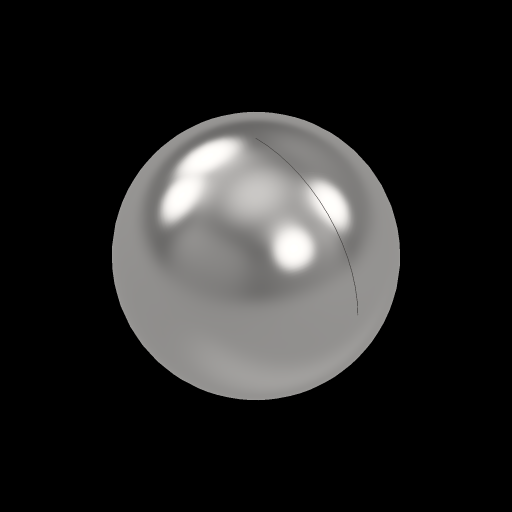
# Autodesk Inventor part: Ball
Saved by Autodesk Inventor 2024 (Build 280153000, 153)
## iProperties
Created: 2023-11-09
Part Number: Ball
Material: Steel, Alloy
Document SubType Name: Modeling
Designer: Admin
Density: 7.73 g/cm^3
Appearance: Semi-Polished
Author: Admin
Autodesk Inventor part; units mm, degrees
ref_plane "YZ Plane" through (0, 0, 0) normal (1, 0, 0) x (0, 1, 0)
ref_plane "XZ Plane" through (0, 0, 0) normal (0, 1, 0) x (-1, 0, 0)
ref_plane "XY Plane" through (0, 0, 0) normal (0, 0, 1) x (1, 0, 0)
sketch "Sketch3" plane through (0, 0, 0) normal (0, 0, 1) x (1, 0, 0)
  arc A0 (4, 0) -> (0, 4) centre (0, 0) ccw
  line L0 (0, 0) -> (4, 0)
  arc A1 (-4, 0) -> (0, -4) centre (0, 0) ccw
  line L1 (-4, 0) -> (0, 0)
  line L2 (0, -6.7598) -> (0, 6.7598) projected
  point P0 (0, 4)
  dimension "d8" = 4
  dimension "d9" = 4
  constraints: 4 end point, 4 point on circle, 2 centre point, 2 coincident, 2 horizontal, 1 point on line
  measures "d8" radius of A0
  measures "d9" radius of A1
extrude "Extrusion2" add sketch "Sketch3" along normal blind 0.01
revolve "Revolution1" add sketch "Sketch3" angle 360 about axis through (0, -10, 0) along (0, 1, 0) contours L0 L2 A0
revolve "Revolution3" add sketch "Sketch3" angle 360 about axis through (0, -10, 0) along (0, 1, 0) contours L2 A1 L1
body "Solid2"
